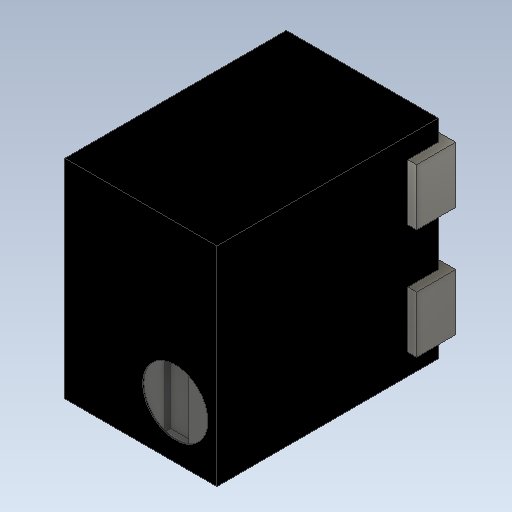
# Autodesk Inventor part: SM42W
Saved by Autodesk Inventor 2020 (Build 240168000, 168)
## iProperties
Created: 2018-04-11
Part Number: SM42W
Material: Generic
Document SubType Name: Modeling
Designer: Alex
Density: 1 g/cm^3
Appearance: Default
Author: Alex
Autodesk Inventor part; units mm, degrees
ref_plane "YZ Plane" through (0, 0, 0) normal (1, 0, 0) x (0, 1, 0)
ref_plane "XZ Plane" through (0, 0, 0) normal (0, 1, 0) x (-1, 0, 0)
ref_plane "XY Plane" through (0, 0, 0) normal (0, 0, 1) x (1, 0, 0)
sketch "Sketch1" plane through (0, 0, 0) normal (0, 0, 1) x (1, 0, 0)
  line L0 (1.75, -2.4) -> (-1.75, -2.4)
  line L1 (-1.75, -2.4) -> (-1.75, 2.4)
  line L2 (-1.75, 2.4) -> (1.75, 2.4)
  line L3 (1.75, 2.4) -> (1.75, -2.4)
  line L4 (1.75, -2.4) -> (-1.75, 2.4) construction
  line L5 (-1.75, -2.4) -> (1.75, 2.4) construction
  point P0 (0, 0)
  dimension "d0" = 3.5
  dimension "d1" = 4.8
  constraints: 12 end point, 2 midpoint, 2 parallel, 1 horizontal, 1 perpendicular
  measures "d0" distance of L1.end L2.end
  measures "d1" distance of L0.end L1.end
extrude "Extrusion1" add sketch "Sketch1" along normal blind 5.1
sketch "Sketch2" plane through (0, 0, 5.1) normal (0, 0, 1) x (1, 0, 0)
  circle A0 centre (0.79, -1.2) radius 0.75
  line L0 (-1.75, 2.4) -> (-1.75, -2.4) projected
  point P0 (0, 0)
  dimension "d4" = 1.5
  dimension "d5" = 1.2
  dimension "d6" = 2.54
  constraints: 1 centre point
  measures "d4" diameter of A0
  measures "d5" vertical distance of A0.centre point (0, 0)
  measures "d6" distance from line of A0.centre L0
extrude "Extrusion2" cut sketch "Sketch2" against normal blind 0.0254
sketch "Sketch3" plane through (0.79, -1.2, 5.0746) normal (0, 0, 1) x (1, 0, 0)
  circle A0 centre (0, 0) radius 0.75 projected
  line L0 (0.28, -0.75) -> (-0.28, -0.75)
  line L1 (-0.28, -0.75) -> (-0.28, 0.75)
  line L2 (-0.28, 0.75) -> (0.28, 0.75)
  line L3 (0.28, 0.75) -> (0.28, -0.75)
  line L4 (0.28, -0.75) -> (-0.28, 0.75) construction
  line L5 (-0.28, -0.75) -> (0.28, 0.75) construction
  point P0 (-0.79, 1.2)
  point P1 (0, 0.75)
  dimension "d9" = 0.56
  constraints: 12 end point, 3 midpoint, 2 parallel, 1 horizontal, 1 perpendicular, 1 vertical alignment, 1 other
  measures "d9" distance between parallel lines of L3 L1
extrude "Extrusion3" cut sketch "Sketch3" against normal blind 0.15 contours L3 A0 L1 | A0 L2 L3 | L3 L0 A0 | A0 L1 L2 | L0 L1 A0
sketch "Sketch4" plane through (0, 0, 0) normal (0, 0, -1) x (-1, 0, 0)
  line L0 (-1.95, 1.92) -> (-0.95, 1.92)
  line L1 (-0.95, 1.92) -> (-0.95, 0.62)
  line L2 (-0.95, 0.62) -> (-1.95, 0.62)
  line L3 (-1.95, 0.62) -> (-1.95, 1.92)
  line L4 (-1.95, -0.62) -> (-0.95, -0.62)
  line L5 (-0.95, -0.62) -> (-0.95, -1.92)
  line L6 (-0.95, -1.92) -> (-1.95, -1.92)
  line L7 (-1.95, -1.92) -> (-1.95, -0.62)
  line L8 (0.95, 0.65) -> (1.95, 0.65)
  line L9 (1.95, 0.65) -> (1.95, -0.65)
  line L10 (1.95, -0.65) -> (0.95, -0.65)
  line L11 (0.95, -0.65) -> (0.95, 0.65)
  line L12 (1.75, -2.4) -> (1.75, 2.4) projected
  line L13 (-1.75, 2.4) -> (-1.75, -2.4) projected
  line L14 (-1.95, 1.27) -> (-0.95, 1.27) construction
  line L15 (-1.95, -1.27) -> (-0.95, -1.27) construction
  point P0 (0, 0)
  point P1 (0.95, 0)
  dimension "d12" = 1
  dimension "d13" = 1.3
  dimension "d14" = 0.2
  dimension "d15" = 0.2
  dimension "d16" = 2.54
  dimension "d17" = 1.27
  constraints: 28 end point, 6 parallel, 5 midpoint, 4 equal length, 3 horizontal, 3 perpendicular, 1 horizontal alignment, 1 point on line, 1 vertical alignment
  measures "d12" distance of L0.start L0.end
  measures "d13" distance of L2.end L0.start
  measures "d14" distance between parallel lines of L12 L9
  measures "d15" distance between parallel lines of L13 L3
  measures "d16" distance between parallel lines of L15 L14
  measures "d17" distance from line of point (0, 0) L14
extrude "Extrusion4" add sketch "Sketch4" along normal blind 0.2 and the other way blind 0.7
equation "\"d15\" = d14"
equation "\"d17\" = 0.5 * d16"
body "Solid1"
